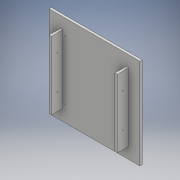
# Autodesk Inventor part: 垃圾桶底板
Saved by Autodesk Inventor 2017 (Build 210142000, 142)
## iProperties
Part Number: 垃圾桶底板
Material: 常规
Document SubType Name: Modeling
Designer: PANDA
Density: 1 g/cm^3
Appearance: 默认
Author: PANDA
Autodesk Inventor part; units mm, degrees
ref_plane "YZ Plane" through (0, 0, 0) normal (1, 0, 0) x (0, 1, 0)
ref_plane "XZ Plane" through (0, 0, 0) normal (0, 1, 0) x (-1, 0, 0)
ref_plane "XY Plane" through (0, 0, 0) normal (0, 0, 1) x (1, 0, 0)
sketch "草图1" plane through (0, 0, 0) normal (0, 1, 0) x (-1, 0, 0)
  line L0 (200, 200) -> (-200, 200)
  line L1 (-200, 200) -> (-200, -200)
  line L2 (-200, -200) -> (200, -200)
  line L3 (200, -200) -> (200, 200)
  point P0 (0, 0)
  dimension "d0" = 400
  dimension "d1" = 400
  constraints: 8 end point, 2 parallel, 1 horizontal, 1 perpendicular
  measures "d0" distance of L2.end L1.end
  measures "d1" distance of L1.end L0.end
extrude "拉伸1" add sketch "草图1" along normal blind 10
sketch "草图2" plane through (0, 10, 0) normal (0, 1, 0) x (1, 0, 0)
  circle A0 centre (130, 130) radius 1.5
  circle A1 centre (-130, 130) radius 1.5
  circle A2 centre (-130, -130) radius 1.5
  point P0 (0, 0)
  constraints: 3 centre point
hole "孔1" at (-130, 10, 130) direction (0, -1, 0) diameter 3 end through all
sketch "草图3" plane through (0, 10, 0) normal (0, 1, 0) x (1, 0, 0)
  circle A0 centre (130, 130) radius 1.5
  point P0 (0, 0)
  constraints: 1 centre point
hole "孔2" at (130, 10, -130) direction (0, -1, 0) diameter 3 end through all
sketch "草图4" plane through (0, 10, 0) normal (0, 1, 0) x (1, 0, 0)
  circle A0 centre (-130, 130) radius 1.5
  point P0 (0, 0)
  constraints: 1 centre point
hole "孔3" at (-130, 10, -130) direction (0, -1, 0) diameter 3 end through all
sketch "草图5" plane through (0, 10, 0) normal (0, 1, 0) x (1, 0, 0)
  circle A0 centre (130, -130) radius 1.5
  point P0 (0, 0)
  constraints: 1 centre point
hole "孔4" at (130, 10, 130) direction (0, -1, 0) diameter 3 end through all
sketch "草图6" plane through (0, 0, 0) normal (0, -1, 0) x (1, 0, 0)
  line L0 (150, 150) -> (-150, 150)
  line L1 (-150, 150) -> (-150, -150)
  line L2 (-150, -150) -> (150, -150)
  line L3 (150, -150) -> (150, 150)
  point P0 (0, 0)
  dimension "d38" = 300
  dimension "d39" = 300
  constraints: 8 end point, 2 parallel, 1 horizontal, 1 perpendicular
  measures "d38" distance of L2.end L1.end
  measures "d39" distance of L1.end L0.end
extrude "拉伸2" add sketch "草图6" along normal blind 50
sketch "草图7" plane through (0, -50, 0) normal (0, -1, 0) x (1, 0, 0)
  line L0 (-150, 150) -> (150, 150) projected
  line L1 (140, 150) -> (-140, 150)
  line L2 (-140, 150) -> (-140, -150)
  line L3 (-140, -150) -> (140, -150)
  line L4 (140, -150) -> (140, 150)
  point P0 (0, 0)
  dimension "d42" = 280
  dimension "d43" = 300
  constraints: 8 end point, 2 parallel, 1 horizontal, 1 perpendicular, 1 point on line
  measures "d42" distance of L3.end L2.end
  measures "d43" distance of L2.end L1.end
extrude "拉伸3" cut sketch "草图7" against normal blind 50
sketch "草图8" plane through (150, 0, 150) normal (1, 0, 0) x (0, 0, -1)
  circle A0 centre (75, -25) radius 2
  point P0 (150, 0)
  constraints: 1 centre point
hole "孔5" at (150, -25, 75) direction (-1, 0, 0) diameter 4 end through all
sketch "草图9" plane through (150, 0, 150) normal (1, 0, 0) x (0, 0, -1)
  circle A0 centre (225, -25) radius 2
  point P0 (150, 0)
  constraints: 1 centre point
hole "孔6" at (150, -25, -75) direction (-1, 0, 0) diameter 4 end through all
